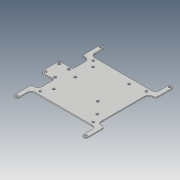
# Autodesk Inventor part: groundPlate
Saved by Autodesk Inventor 2018 (Build 220112000, 112)
## iProperties
Created: 2020-02-04
Part Number: groundPlate
Material: Generic
Document SubType Name: Modeling
Designer: anirudh.bali
Density: 1 g/cm^3
Appearance: Default
Author: anirudh.bali
Autodesk Inventor part; units mm, degrees
ref_plane "YZ Plane" through (0, 0, 0) normal (1, 0, 0) x (0, 1, 0)
ref_plane "XZ Plane" through (0, 0, 0) normal (0, 1, 0) x (-1, 0, 0)
ref_plane "XY Plane" through (0, 0, 0) normal (0, 0, 1) x (1, 0, 0)
sketch "Sketch7" plane through (0, 0, 0) normal (0, 1, 0) x (-1, 0, 0)
  line L0 (93.98, -93.98) -> (0, -93.98)
  line L1 (0, -87.376) -> (0, -6.604)
  circle A0 centre (101.4857, 19.3548) radius 1.85
  circle A1 centre (101.4857, 19.3548) radius 1.85
  circle A2 centre (-7.5057, 19.3548) radius 1.85
  circle A3 centre (-7.5057, 19.3548) radius 1.85
  circle A4 centre (-7.5057, -113.3348) radius 1.85
  circle A5 centre (101.4857, -113.3348) radius 1.85
  circle A6 centre (101.4857, -113.3348) radius 1.85
  arc A7 (104.7877, 19.3548) -> (98.1837, 19.3548) centre (101.4857, 19.3548) ccw
  arc A8 (-4.2037, 19.3548) -> (-10.8077, 19.3548) centre (-7.5057, 19.3548) ccw
  arc A9 (-10.8077, -113.3348) -> (-4.2037, -113.3348) centre (-7.5057, -113.3348) ccw
  arc A10 (98.1837, -113.3348) -> (104.7877, -113.3348) centre (101.4857, -113.3348) ccw
  line L2 (98.1837, 19.3548) -> (98.1837, 0)
  line L3 (98.1837, 0) -> (93.98, 0)
  line L4 (104.7877, 19.3548) -> (104.7877, 0)
  line L5 (104.7877, 0) -> (104.7877, -6.604)
  line L6 (104.7877, -6.604) -> (93.98, -6.604)
  arc A11 (98.1837, -113.3348) -> (104.7877, -113.3348) centre (101.4857, -113.3348) ccw
  line L7 (98.1837, -113.3348) -> (98.1837, -93.98)
  line L8 (98.1837, -93.98) -> (93.98, -93.98)
  line L9 (104.7877, -113.3348) -> (104.7877, -93.98)
  line L10 (104.7877, -93.98) -> (104.7877, -87.376)
  line L11 (104.7877, -87.376) -> (93.98, -87.376)
  arc A12 (-4.2037, 19.3548) -> (-10.8077, 19.3548) centre (-7.5057, 19.3548) ccw
  line L12 (-4.2037, 19.3548) -> (-4.2037, 0)
  line L13 (-4.2037, 0) -> (0, 0)
  line L14 (-10.8077, 19.3548) -> (-10.8077, 0)
  line L15 (-10.8077, 0) -> (-10.8077, -6.604)
  line L16 (-10.8077, -6.604) -> (0, -6.604)
  arc A13 (-10.8077, -113.3348) -> (-4.2037, -113.3348) centre (-7.5057, -113.3348) ccw
  line L17 (-4.2037, -113.3348) -> (-4.2037, -93.98)
  line L18 (-10.8077, -113.3348) -> (-10.8077, -93.98)
  line L19 (-10.8077, -87.376) -> (0, -87.376)
  line L20 (-4.2037, -93.98) -> (0, -93.98)
  line L21 (-10.8077, -93.98) -> (-10.8077, -87.376)
  circle A14 centre (88.9, -5.08) radius 1.75
  circle A15 centre (88.9, -88.9) radius 1.75
  circle A16 centre (5.08, -5.08) radius 1.75
  circle A17 centre (5.08, -88.9) radius 1.75
  line L22 (98.1837, 0) -> (-4.2037, 0)
  circle A18 centre (80.64, -80.3026) radius 1.75
  circle A19 centre (80.64, -52.1326) radius 1.75
  circle A20 centre (28.58, -85.1226) radius 1.75
  circle A21 centre (29.83, -36.8026) radius 1.75
  circle A22 centre (81.275, -18.8574) radius 1.75
  circle A23 centre (12.705, -18.8574) radius 1.75
  line L23 (88.9, -5.08) -> (90.65, -5.08) construction
  circle A24 centre (111.661, -36.195) radius 2
  circle A25 centre (111.661, -57.785) radius 2
  circle A26 centre (96.421, -36.195) radius 2
  circle A27 centre (96.421, -57.785) radius 2
  line L24 (93.98, -32.484) -> (114.102, -32.484)
  line L25 (114.102, -32.484) -> (115.372, -32.484)
  line L26 (115.372, -32.484) -> (115.372, -60.226)
  line L27 (115.372, -60.226) -> (115.372, -61.496)
  line L28 (115.372, -61.496) -> (93.98, -61.496)
  line L29 (93.98, -61.496) -> (93.98, -87.376)
  line L30 (93.98, -6.604) -> (93.98, -32.484)
  point P0 (-2.54, 0.1)
  constraints: 62 end point, 28 centre point, 14 point on circle, 12 coincident, 6 point on line, 3 perpendicular, 3 vertical, 2 horizontal
extrude "Extrusion5" add sketch "Sketch7" along normal blind 1.5875
fillet "Fillet8" radius 6.35 8 edges at (-98.1837, 0.7937, 0) (-93.98, 0.7937, -6.604) (4.2037, 0.7937, 0) (0, 0.7937, -6.604) (0, 0.7937, -87.376) (4.2037, 0.7937, -93.98) (-93.98, 0.7937, -87.376) (-98.1837, 0.7937, -93.98)
fillet "Fillet9" radius 3.175 8 edges at (-104.7877, 0.7937, -6.604) (-115.372, 0.7937, -32.484) (-93.98, 0.7937, -32.484) (-93.98, 0.7937, -61.496) (-115.372, 0.7937, -61.496) (-104.7877, 0.7937, -87.376) (10.8077, 0.7937, -87.376) (10.8077, 0.7937, -6.604)
body "Solid3"
